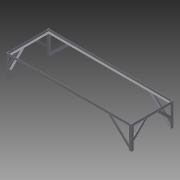
# Autodesk Inventor part: Burner_Stand
Saved by Autodesk Inventor 2014 (Build 180170000, 170)
## iProperties
Created: 2016-08-25
Part Number: Burner_Stand
Material: Generic
Document SubType Name: Modeling
Designer: jmw3
Density: 1 g/cm^3
Appearance: Default
Author: jmw3
Autodesk Inventor part; units mm, degrees
ref_plane "YZ Plane" through (0, 0, 0) normal (1, 0, 0) x (0, 1, 0)
ref_plane "XZ Plane" through (0, 0, 0) normal (0, 1, 0) x (-1, 0, 0)
ref_plane "XY Plane" through (0, 0, 0) normal (0, 0, 1) x (1, 0, 0)
sketch "Sketch1" plane through (0, 0, 0) normal (0, 1, 0) x (-1, 0, 0)
  line L0 (0, -471.17) -> (0, 471.17) projected
  line L1 (1409.065, 0) -> (-1409.065, 0) projected
  line L2 (-1003.3, 333.375) -> (1003.3, 333.375)
  line L3 (1003.3, 333.375) -> (1003.3, -333.375)
  line L4 (1003.3, -333.375) -> (-1003.3, -333.375)
  line L5 (-1003.3, -333.375) -> (-1003.3, 333.375)
  line L6 (-968.375, 298.45) -> (968.375, 298.45)
  line L7 (968.375, 298.45) -> (968.375, -298.45)
  line L8 (968.375, -298.45) -> (-968.375, -298.45)
  line L9 (-968.375, -298.45) -> (-968.375, 298.45)
  line L10 (-1006.475, 336.55) -> (1006.475, 336.55)
  line L11 (1006.475, 336.55) -> (1006.475, -336.55)
  line L12 (1006.475, -336.55) -> (-1006.475, -336.55)
  line L13 (-1006.475, -336.55) -> (-1006.475, 336.55)
  point P0 (0, 0)
  dimension "d0" = 2006.6
  dimension "d1" = 666.75
  dimension "d2" = 596.9
  dimension "d3" = 1936.75
  dimension "d4" = 3.175
  dimension "d5" = 3.175
  constraints: 24 end point, 6 parallel, 3 horizontal, 3 perpendicular, 6 other
  measures "d0" distance between parallel lines of L3 L5
  measures "d1" distance between parallel lines of L4 L2
  measures "d2" distance between parallel lines of L8 L6
  measures "d3" distance between parallel lines of L7 L9
  measures "d4" distance between parallel lines of L5 L13
  measures "d5" distance between parallel lines of L4 L12
extrude "Extrusion1" add sketch "Sketch1" against normal blind 3.175 contours L12 L13 L1 L5 L4 L0 | L0 L4 L3 L1 L11 L12 | L4 L5 L1 L9 L8 L0 | L0 L8 L7 L1 L3 L4 | L1 L3 L2 L0 L10 L11 | L13 L10 L0 L2 L5 L1 | L1 L7 L6 L0 L2 L3 | L5 L2 L0 L6 L9 L1
extrude "Extrusion2" add sketch "Sketch1" along normal blind 34.925 contours L12 L13 L1 L5 L4 L0 | L0 L4 L3 L1 L11 L12 | L1 L3 L2 L0 L10 L11 | L13 L10 L0 L2 L5 L1
sketch "Sketch2" plane through (0, 34.925, 0) normal (0, 1, 0) x (1, 0, 0)
  line L0 (1006.475, -336.55) -> (1006.475, 336.55) projected
  line L1 (1006.475, 336.55) -> (-1006.475, 336.55) projected
  line L2 (971.55, 336.55) -> (1006.475, 336.55)
  line L3 (1006.475, 339.725) -> (971.55, 339.725)
  line L4 (971.55, 339.725) -> (971.55, 336.55)
  line L5 (1006.475, 339.725) -> (1009.65, 339.725)
  line L6 (1009.65, 339.725) -> (1009.65, 301.625)
  line L7 (1009.65, 301.625) -> (1006.475, 301.625)
  line L8 (1006.475, 301.625) -> (1006.475, 336.55)
  point P0 (0, 0)
  dimension "d10" = 3.175
  dimension "d15" = 3.175
  dimension "d41" = 38.1
  dimension "d42" = 38.1
  constraints: 14 end point, 3 parallel, 2 horizontal, 1 collinear, 1 perpendicular, 1 point on line
  measures "d10" distance between parallel lines of L2 L3
  measures "d15" distance between parallel lines of L0 L6
  measures "d41" distance between parallel lines of L6 L4
  measures "d42" distance between parallel lines of L3 L7
extrude "Extrusion3" add sketch "Sketch2" against normal blind 381
sketch "Sketch4" plane through (1006.475, -3.175, 336.55) normal (1, 0, 0) x (0, 0, -1)
  line L0 (638.175, 0) -> (0, 0) projected
  line L1 (447.479, 24.9105) -> (420.7746, -2.2646)
  line L2 (420.7746, -2.2646) -> (638.175, -215.9)
  line L3 (638.175, -215.9) -> (638.175, -162.483)
  line L4 (638.175, -162.483) -> (447.479, 24.9105)
  line L5 (638.175, 38.1) -> (638.175, -342.9) projected
  line L6 (676.275, -342.9) -> (638.175, -342.9) projected
  line L7 (422.9999, 0) -> (638.175, -211.4486)
  line L8 (422.9999, 0) -> (420.7746, -2.2646)
  line L9 (420.7746, -2.2646) -> (638.175, -215.9)
  line L10 (638.175, -215.9) -> (638.175, -211.4486)
  line L11 (638.175, -211.4486) -> (422.9999, 0)
  point P0 (336.55, 3.175)
  dimension "d23" = 38.1
  dimension "d24" = 304.8
  dimension "d25" = 127
  dimension "d28" = 3.175
  constraints: 18 end point, 4 perpendicular, 3 parallel, 3 point on line, 2 collinear
  measures "d23" distance of L1.start L1.end
  measures "d24" distance from line of L2.end L1
  measures "d25" distance from line of L6 L2.end
  measures "d28" distance between parallel lines of L2 L7
extrude "Extrusion5" add sketch "Sketch4" against normal blind 34.925 contours L7 L3 L2 L1
extrude "Extrusion6" add sketch "Sketch4" along normal blind 3.175 contours L4 L3 L7 L0 | L0 L1 L4 | L7 L3 L2 L1
sketch "Sketch5" plane through (1009.65, 34.925, -339.725) normal (0, 0, -1) x (-1, 0, 0)
  line L0 (38.1, -381) -> (0, -381) projected
  line L1 (38.1, 0) -> (38.1, -381) projected
  line L2 (38.1, 0) -> (38.1, -38.1) projected
  line L3 (2016.125, -38.1) -> (38.1, -38.1) projected
  line L4 (2016.125, 0) -> (2016.125, -38.1) projected
  line L5 (38.1, 0) -> (2016.125, 0) projected
  line L6 (38.1, -355.6) -> (369.2808, -40.3999)
  line L7 (369.2808, -40.3999) -> (343.0141, -12.8015)
  line L8 (343.0141, -12.8015) -> (38.1, -303.0024)
  line L9 (38.1, -303.0024) -> (38.1, -355.6)
  line L10 (367.0919, -38.1) -> (38.1, -351.2169)
  point P0 (1009.65, -34.925)
  dimension "d33" = 38.1
  dimension "d34" = 25.4
  dimension "d35" = 3.175
  dimension "d36" = 457.2
  constraints: 10 end point, 5 point on line, 3 perpendicular, 1 parallel
  measures "d33" distance of L6.end L7.end
  measures "d34" distance from line of L0 L6.start
  measures "d35" distance between parallel lines of L6 L10
  measures "d36" distance from line of L6.start L7
extrude "Extrusion7" add sketch "Sketch5" against normal blind 3.175 contours L8 L3 L10 L1 | L8 L7 L3 | L10 L7 L6 L1
extrude "Extrusion8" add sketch "Sketch5" against normal blind 38.1 contours L10 L7 L6 L1
mirror "Mirror1" about plane through (0, 0, 0) normal (0, 0, 1) of "Extrusion8", "Extrusion7", "Extrusion6", "Extrusion5", "Extrusion3"
mirror "Mirror2" about plane through (0, 0, 0) normal (1, 0, 0) of "Extrusion8", "Extrusion7", "Extrusion6", "Extrusion5", "Extrusion3", "Mirror1"
body "Solid1"
